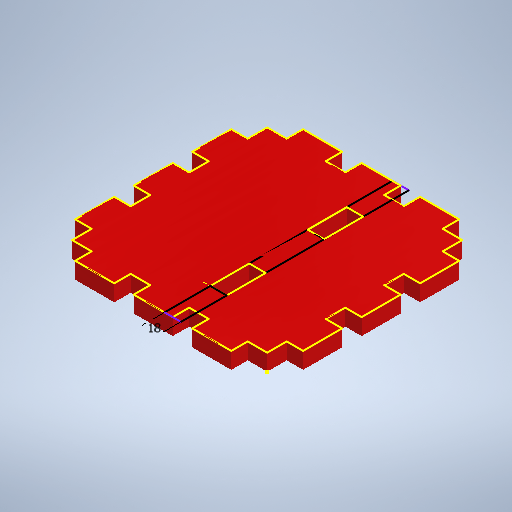
# Autodesk Inventor part: 3
Saved by Autodesk Inventor 2025.3 (Build 293356000, 356)
## iProperties
Created: 2025-12-22
Part Number: 3
Material: Generic
Document SubType Name: Sheet Metal
Designer: Balint
Density: 1 g/cm^3
Sheet Metal Rule: Default_mm
Appearance: Default
Flat Pattern Width: 25 cm
Flat Pattern Length: 25 cm
Flat Pattern Area: 625 cm^2
Sheet Metal Width: 250.000 mm
Sheet Metal Length: 250.000 mm
Sheet Metal Area: 62500.000 mm^2
Author: Balint
Autodesk Inventor part; units mm, degrees
ref_plane "YZ Plane" through (0, 0, 0) normal (1, 0, 0) x (0, 1, 0)
ref_plane "XZ Plane" through (0, 0, 0) normal (0, 1, 0) x (-1, 0, 0)
ref_plane "XY Plane" through (0, 0, 0) normal (0, 0, 1) x (1, 0, 0)
sketch "Sketch1" plane through (0, 0, 0) normal (0, 1, 0) x (-1, 0, 0)
  line L0 (0, 0) -> (250, 0)
  line L1 (250, 0) -> (250, -250)
  line L2 (250, -250) -> (0, -250)
  line L3 (0, -250) -> (0, 0)
  line L4 (232, -232) -> (232, -18)
  line L5 (232, -232) -> (18, -232)
  line L6 (18, -232) -> (232, -232)
  line L7 (250, -18) -> (250, -39.4)
  line L8 (250, -39.4) -> (232, -39.4)
  line L9 (232, -39.4) -> (232, -18)
  line L10 (232, -103.6) -> (250, -103.6)
  line L11 (250, -82.2) -> (232, -82.2)
  line L12 (232, -82.2) -> (232, -103.6)
  line L13 (250, -167.8) -> (232, -167.8)
  line L14 (232, -146.4) -> (250, -146.4)
  line L15 (250, -210.6) -> (232, -210.6)
  line L16 (0, 0) -> (0, -18)
  line L17 (232, -18) -> (232, 0)
  line L18 (0, -39.4) -> (18, -39.4)
  line L19 (0, -82.2) -> (18, -82.2)
  line L20 (18, -103.6) -> (0, -103.6)
  line L21 (18, -146.4) -> (0, -146.4)
  line L22 (0, -167.8) -> (18, -167.8)
  line L23 (0, -210.6) -> (18, -210.6)
  line L24 (39.4, -250) -> (39.4, -232)
  line L25 (82.2, -250) -> (82.2, -232)
  line L26 (103.6, -232) -> (103.6, -250)
  line L27 (146.4, -232) -> (146.4, -250)
  line L28 (167.8, -250) -> (167.8, -232)
  line L29 (210.6, -250) -> (210.6, -232)
  line L30 (146.4, 0) -> (146.4, -18)
  line L31 (103.6, 0) -> (103.6, -18)
  line L32 (82.2, -18) -> (82.2, 0)
  line L33 (39.4, -18) -> (39.4, 0)
  line L34 (167.8, -18) -> (167.8, 0)
  line L35 (210.6, -18) -> (210.6, 0)
  line L36 (232, -18) -> (18, -18)
  line L37 (18, -18) -> (18, -232)
  point P0 (0, -146.4)
  point P1 (18, -232)
  dimension "d0" = 250
  dimension "d1" = 250
  dimension "d4" = 21.4
  measures "d0" distance of L1.end L2.end
  measures "d1" distance of L0.end L1.end
  measures "d4" distance of L7.start L7.end
extrude "Plate2" add sketch "Sketch1" along normal blind 18 contours L0 L32 L36 L33 | L36 L4 L5 L37 | L18 L37 L19 L3 | L0 L30 L36 L31 | L20 L37 L21 L3 | L0 L35 L36 L34 | L22 L37 L23 L3 | L8 L1 L11 L4 | L24 L5 L25 L2 | L10 L1 L14 L4 | L26 L5 L27 L2 | L13 L1 L15 L4 | L28 L5 L29 L2
sketch "Sketch2" plane through (0, 18, 0) normal (0, 1, 0) x (1, 0, 0)
  line L0 (0, 103.6) -> (0, 146.4) projected
  line L1 (-103.6, 18) -> (-82.2, 18) projected
  line L2 (-82.2, 232) -> (-103.6, 232) projected
  line L3 (-103.6, 18) -> (-103.6, 232)
  line L4 (-103.6, 18) -> (-103.6, 125)
  line L5 (-94.6, 50.1) -> (-112.6, 50.1)
  line L6 (-112.6, 50.1) -> (-112.6, 92.9)
  line L7 (-112.6, 92.9) -> (-94.6, 92.9)
  line L8 (-94.6, 92.9) -> (-94.6, 50.1)
  line L9 (-94.6, 50.1) -> (-112.6, 92.9) construction
  line L10 (-112.6, 50.1) -> (-94.6, 92.9) construction
  line L11 (-103.6, 232) -> (-103.6, 125)
  line L12 (-103.6, 125) -> (-103.6, 178.5)
  line L13 (-94.6, 199.9) -> (-112.6, 199.9)
  line L14 (-112.6, 199.9) -> (-112.6, 157.1)
  line L15 (-112.6, 157.1) -> (-94.6, 157.1)
  line L16 (-94.6, 157.1) -> (-94.6, 199.9)
  line L17 (-94.6, 199.9) -> (-112.6, 157.1) construction
  line L18 (-112.6, 199.9) -> (-94.6, 157.1) construction
  point P0 (0, 0)
  point P1 (-103.6, 71.5)
  dimension "d7" = 18
  dimension "d8" = 42.8
  dimension "d9" = 42.8
  constraints: 32 end point, 7 midpoint, 4 parallel, 2 horizontal, 2 perpendicular, 1 collinear, 1 vertical
  measures "d7" distance of L6.end L7.end
  measures "d8" distance of L5.end L6.end
  measures "d9" distance of L14.end L13.end
extrude "Cut1" cut sketch "Sketch2" against normal blind 18
sketch "Sketch3" plane through (0, 18, 0) normal (0, 1, 0) x (1, 0, 0)
  line L0 (-112.6, 50.1) -> (-94.6, 50.1)
  line L1 (-94.6, 50.1) -> (-94.6, 0)
  line L2 (-94.6, 0) -> (-112.6, 0)
  line L3 (-112.6, 0) -> (-112.6, 50.1)
  line L4 (-94.6, 199.9) -> (-94.6, 157.1) projected
  line L5 (-94.6, 157.1) -> (-112.6, 157.1) projected
  line L6 (-112.6, 157.1) -> (-112.6, 199.9) projected
  line L7 (-112.6, 199.9) -> (-94.6, 199.9) projected
  line L8 (-112.6, 50.1) -> (-112.6, 92.9) projected
  line L9 (-112.6, 92.9) -> (-94.6, 92.9) projected
  line L10 (-94.6, 92.9) -> (-94.6, 50.1) projected
  line L11 (-94.6, 50.1) -> (-112.6, 50.1) projected
  line L12 (-250, 82.2) -> (-232, 82.2) projected
  line L13 (-250, 39.4) -> (-250, 82.2) projected
  line L14 (-232, 39.4) -> (-250, 39.4) projected
  line L15 (-232, 18) -> (-232, 39.4) projected
  line L16 (-210.6, 18) -> (-232, 18) projected
  line L17 (-210.6, 0) -> (-210.6, 18) projected
  line L18 (-167.8, 0) -> (-210.6, 0) projected
  line L19 (-167.8, 18) -> (-167.8, 0) projected
  line L20 (-146.4, 18) -> (-167.8, 18) projected
  line L21 (-146.4, 0) -> (-146.4, 18) projected
  line L22 (-103.6, 0) -> (-146.4, 0) projected
  line L23 (-103.6, 18) -> (-103.6, 0) projected
  line L24 (-82.2, 18) -> (-103.6, 18) projected
  line L25 (-82.2, 0) -> (-82.2, 18) projected
  line L26 (-39.4, 0) -> (-82.2, 0) projected
  line L27 (-39.4, 18) -> (-39.4, 0) projected
  line L28 (-18, 18) -> (-39.4, 18) projected
  line L29 (-18, 39.4) -> (-18, 18) projected
  line L30 (0, 39.4) -> (-18, 39.4) projected
  line L31 (0, 82.2) -> (0, 39.4) projected
  line L32 (-18, 82.2) -> (0, 82.2) projected
  line L33 (-18, 103.6) -> (-18, 82.2) projected
  line L34 (0, 103.6) -> (-18, 103.6) projected
  line L35 (0, 146.4) -> (0, 103.6) projected
  line L36 (-18, 146.4) -> (0, 146.4) projected
  line L37 (-18, 167.8) -> (-18, 146.4) projected
  line L38 (0, 167.8) -> (-18, 167.8) projected
  line L39 (0, 210.6) -> (0, 167.8) projected
  line L40 (-18, 210.6) -> (0, 210.6) projected
  line L41 (-18, 232) -> (-18, 210.6) projected
  line L42 (-39.4, 232) -> (-18, 232) projected
  line L43 (-39.4, 250) -> (-39.4, 232) projected
  line L44 (-82.2, 250) -> (-39.4, 250) projected
  line L45 (-82.2, 232) -> (-82.2, 250) projected
  line L46 (-103.6, 232) -> (-82.2, 232) projected
  line L47 (-103.6, 250) -> (-103.6, 232) projected
  line L48 (-146.4, 250) -> (-103.6, 250) projected
  line L49 (-146.4, 232) -> (-146.4, 250) projected
  line L50 (-167.8, 232) -> (-146.4, 232) projected
  line L51 (-167.8, 250) -> (-167.8, 232) projected
  line L52 (-210.6, 250) -> (-167.8, 250) projected
  line L53 (-210.6, 232) -> (-210.6, 250) projected
  line L54 (-232, 232) -> (-210.6, 232) projected
  line L55 (-232, 210.6) -> (-232, 232) projected
  line L56 (-250, 210.6) -> (-232, 210.6) projected
  line L57 (-250, 167.8) -> (-250, 210.6) projected
  line L58 (-232, 167.8) -> (-250, 167.8) projected
  line L59 (-232, 146.4) -> (-232, 167.8) projected
  line L60 (-250, 146.4) -> (-232, 146.4) projected
  line L61 (-250, 103.6) -> (-250, 146.4) projected
  line L62 (-232, 103.6) -> (-250, 103.6) projected
  line L63 (-232, 82.2) -> (-232, 103.6) projected
  line L64 (-112.6, 50.1) -> (-94.6, 50.1)
  line L65 (-94.6, 50.1) -> (-94.6, 92.9)
  line L66 (-94.6, 92.9) -> (-112.6, 92.9)
  line L67 (-112.6, 92.9) -> (-112.6, 50.1)
  line L68 (-94.6, 92.9) -> (-112.6, 92.9)
  line L69 (-112.6, 92.9) -> (-112.6, 157.1)
  line L70 (-112.6, 157.1) -> (-94.6, 157.1)
  line L71 (-94.6, 157.1) -> (-94.6, 92.9)
  line L72 (-112.6, 157.1) -> (-112.6, 199.9) projected
  line L73 (-94.6, 157.1) -> (-112.6, 157.1)
  line L74 (-112.6, 157.1) -> (-112.6, 199.9)
  line L75 (-112.6, 199.9) -> (-94.6, 199.9)
  line L76 (-94.6, 199.9) -> (-94.6, 157.1)
  line L77 (-112.6, 199.9) -> (-94.6, 199.9)
  line L78 (-94.6, 199.9) -> (-94.6, 250)
  line L79 (-94.6, 250) -> (-112.6, 250)
  line L80 (-112.6, 250) -> (-112.6, 199.9)
  point P0 (0, 0)
  dimension "d12" = 18
  constraints: 40 end point, 10 parallel, 5 horizontal, 5 perpendicular, 1 point on line
  measures "d12" distance of L1.end L2.end
equation "\"d10\" = Thickness"
equation "\"d5\" = Thickness"
equation "\"BendRadius\" = Thickness"
equation "\"BendReliefWidth\" = Thickness"
equation "\"BendReliefDepth\" = 0.5 * Thickness"
equation "\"CornerReliefSize\" = 4 * Thickness"
equation "\"MinimumRemnant\" = 2 * Thickness"
equation "\"TransitionRadius\" = BendRadius"
equation "\"JacobiRadiusSize\" = BendRadius"
equation "\"GapSize\" = Thickness"
equation "\"Thickness\" = 18"
body "Solid2"
